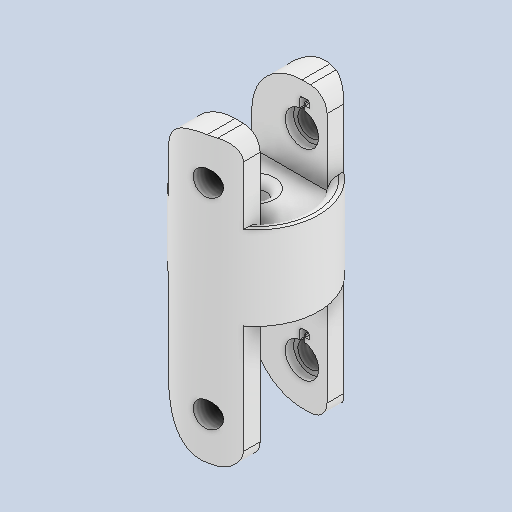
# Autodesk Inventor part: Thumb_1
Saved by Autodesk Inventor 2022 (Build 260153000, 153)
## iProperties
Created: 2023-01-15
Part Number: Thumb_1
Material: ABS Plastic
Document SubType Name: Modeling
Designer: 48735
Density: 1.06 g/cm^3
Appearance: Smooth - White
Author: 48735
Autodesk Inventor part; units mm, degrees
ref_plane "YZ Plane" through (0, 0, 0) normal (1, 0, 0) x (0, 1, 0)
ref_plane "XZ Plane" through (0, 0, 0) normal (0, 1, 0) x (-1, 0, 0)
ref_plane "XY Plane" through (0, 0, 0) normal (0, 0, 1) x (1, 0, 0)
sketch "Sketch1" plane through (0, 0, 0) normal (0, 1, 0) x (-1, 0, 0)
  circle A0 centre (0, 0) radius 7.5
  line L0 (0, -4) -> (6.3443, -4)
  line L1 (0, -4) -> (-6.3443, -4)
  line L2 (0, 4) -> (-6.3443, 4)
  line L3 (0, 4) -> (6.3443, 4)
  line L4 (7.5, 0) -> (4.5, 0)
  line L5 (4.5, 0) -> (4.5, 6)
  line L6 (4.5, 0) -> (4.5, -6)
  line L7 (-7.5, 0) -> (-4.5, 0)
  line L8 (-4.5, 0) -> (-4.5, 6)
  line L9 (-4.5, 0) -> (-4.5, -6)
  point P0 (-4.5, -4)
  point P1 (4.5, -4)
  point P2 (-4.5, 4)
  point P3 (4.5, 4)
  dimension "d5" = 3
  dimension "d6" = 3
  constraints: 20 end point, 5 point on line, 2 parallel, 2 perpendicular, 1 coincident, 12 other
  measures "d5" distance of L4.start L4.end
  measures "d6" distance of L7.start L7.end
extrude "Extrusion1" add sketch "Sketch1" along normal blind 15 contours L5 L3 L2 L8 A0 | A0 L9 L1 L0 L6
sketch "Sketch2" plane through (0, 15, 0) normal (0, 1, 0) x (1, 0, 0)
  circle A0 centre (0, 0) radius 7.5
  circle A1 centre (0, 0) radius 1.25
  dimension "d7" = 2.5
  constraints: 2 centre point, 2 coincident
  measures "d7" diameter of A1
extrude "Extrusion2" add sketch "Sketch2" along normal blind 10
sketch "Sketch3" plane through (-4.5, 0, -4) normal (0, 0, 1) x (1, 0, 0)
  circle A0 centre (3.25, 12.5) radius 1.25
  point P0 (4.5, 0)
  constraints: 1 centre point
extrude "Extrusion3" add sketch "Sketch3" along normal blind 4
chamfer "Chamfer1" distance 0.25 distance2 1.25 1 edges at (-2.5, 12.5, 0) measured on face at (-0.9381, 12.7763, 0)
sketch "Sketch4" plane through (4.5, 0, 4) normal (0, 0, -1) x (-1, 0, 0)
  circle A0 centre (5.75, 12.5) radius 1.25
  point P0 (4.5, 0)
  constraints: 1 centre point
extrude "Extrusion4" add sketch "Sketch4" along normal blind 4
fillet "Fillet1" radius 6 2 edges at (-4.5, 0, 5) (-4.5, 0, -5)
fillet "Fillet2" radius 2 2 edges at (4.5, 0, 5) (4.5, 0, -5)
chamfer "Chamfer2" distance 1 angle 45 1 edges at (-7.5, 15, 0)
chamfer "Chamfer3" distance 0.25 distance2 1.25 1 edges at (0, 12.5, 0) measured on face at (-2.3949, 12.3205, 0)
sketch "Sketch5" plane through (4.5, 15, 4) normal (0, 0, -1) x (-1, 0, 0)
  arc A0 (3, -15) -> (9, -9) centre (3, -9) ccw projected
  line L0 (3, -15) -> (3, -10)
  point P0 (4.5, -15)
  dimension "d29" = 5
  constraints: 2 end point, 1 vertical
  measures "d29" distance of L0.start L0.end
hole "Hole1" at (1.5, 5, 4) direction (0, 0, 1) diameter 3 depth 5 counterbore diameter 4 counterbore depth 1
sketch "Sketch6" plane through (-4.5, 15, -4) normal (0, 0, 1) x (1, 0, 0)
  circle A0 centre (6, -10) radius 1.75 projected
  line L0 (6, -10) -> (7.75, -10)
  point P0 (4.5, -15)
  constraints: 2 end point, 1 horizontal, 1 horizontal alignment, 1 other
hole "Hole2" at (1.5, 5, -4) direction (0, 0, -1) diameter 3 depth 5 tip angle 118 counterbore diameter 4 counterbore depth 1
sketch "Sketch7" plane through (4.5, 15, 4) normal (0, 0, -1) x (-1, 0, 0)
  circle A0 centre (3, -10) radius 1.75 projected
  line L0 (2.75, -7.25) -> (2.75, -10)
  line L1 (2.75, -10) -> (3, -10)
  line L2 (3, -10) -> (3.25, -10)
  line L3 (3.25, -10) -> (3.25, -7)
  arc A1 (3.25, -7) -> (3, -6.75) centre (3, -7) ccw
  line L4 (3, -6.75) -> (2.5, -6.75)
  line L5 (2.5, -6.75) -> (2.375, -6.75)
  arc A2 (2.375, -6.75) -> (2.125, -7) centre (2.375, -7) ccw
  line L6 (2.125, -7) -> (2.125, -7.5)
  line L7 (2.125, -7.5) -> (2.625, -7.5)
  line L8 (2.625, -7.5) -> (2.625, -7.25)
  line L9 (2.625, -7.25) -> (2.75, -7.25)
  circle A3 centre (3, -10) radius 1.75
  line L10 (2.75, -7.25) -> (2.75, -10)
  line L11 (2.75, -10) -> (3, -10)
  line L12 (3, -10) -> (3.25, -10)
  line L13 (3.25, -10) -> (3.25, -7)
  arc A4 (3.25, -7) -> (3, -6.75) centre (3, -7) ccw
  line L14 (3, -6.75) -> (2.5, -6.75)
  line L15 (2.5, -6.75) -> (2.375, -6.75)
  arc A5 (2.375, -6.75) -> (2.125, -7) centre (2.375, -7) ccw
  line L16 (2.125, -7) -> (2.125, -7.5)
  line L17 (2.125, -7.5) -> (2.625, -7.5)
  line L18 (2.625, -7.5) -> (2.625, -7.25)
  line L19 (2.625, -7.25) -> (2.75, -7.25)
  point P0 (4.5, -15)
  point P1 (4.5, -15)
  constraints: 40 end point, 8 perpendicular, 8 point on circle, 6 tangent, 5 centre point, 4 horizontal, 2 point on line, 2 vertical
sketch "Sketch8" plane through (-4.5, 15, -4) normal (0, 0, 1) x (1, 0, 0)
  circle A0 centre (6, -10) radius 1.75
  line L0 (5.75, -8.2679) -> (5.75, -10)
  line L1 (5.75, -10) -> (6, -10)
  line L2 (6, -10) -> (6.25, -10)
  line L3 (6.25, -10) -> (6.25, -7.25)
  line L4 (5.75, -7.25) -> (5.75, -10)
  line L5 (5.75, -10) -> (6, -10)
  line L6 (6, -10) -> (6.25, -10)
  line L7 (6.25, -10) -> (6.25, -7.25)
  circle A1 centre (6, -10) radius 1.75 projected
  circle A2 centre (6, -10) radius 1.75
  line L8 (6.25, -7.25) -> (6.25, -10)
  line L9 (6.25, -10) -> (6, -10)
  line L10 (6, -10) -> (5.75, -10)
  line L11 (5.75, -10) -> (5.75, -7)
  line L12 (6, -6.75) -> (6.5, -6.75)
  line L13 (6.5, -6.75) -> (6.625, -6.75)
  arc A3 (6.875, -7) -> (6.625, -6.75) centre (6.625, -7) ccw
  line L14 (6.875, -7) -> (6.875, -7.5)
  line L15 (6.875, -7.5) -> (6.375, -7.5)
  line L16 (6.375, -7.5) -> (6.375, -7.25)
  line L17 (6.375, -7.25) -> (6.25, -7.25)
  line L18 (6.25, -7.25) -> (6.25, -10)
  line L19 (6.25, -10) -> (6, -10)
  line L20 (6, -10) -> (5.75, -10)
  line L21 (5.75, -10) -> (5.75, -7)
  arc A4 (6, -6.75) -> (5.75, -7) centre (6, -7) ccw
  line L22 (6, -6.75) -> (6.5, -6.75)
  line L23 (6.5, -6.75) -> (6.625, -6.75)
  arc A5 (6.875, -7) -> (6.625, -6.75) centre (6.625, -7) ccw
  line L24 (6.875, -7) -> (6.875, -7.5)
  line L25 (6.875, -7.5) -> (6.375, -7.5)
  line L26 (6.375, -7.5) -> (6.375, -7.25)
  line L27 (6.375, -7.25) -> (6.25, -7.25)
  point P0 (4.5, -15)
  point P1 (4.5, -15)
  point P2 (4.5, -15)
  point P3 (6.25, -8.2679)
  constraints: 56 end point, 6 point on circle, 4 centre point, 4 perpendicular, 4 point on line, 3 other
extrude "Extrusion5" cut sketch "Sketch7" against normal blind 1 contours L3 L2 L1 L0 A0 | A0 L0 L9 L8 L7 L6 A2 L5 L4 A1 L3 picked at (3.1667, -9.4226)
extrude "Extrusion6" cut sketch "Sketch8" against normal blind 1 contours L4 L11 A4 L12 L13 A3 L14 L15 L16 L17 L3 A0
sketch "Sketch9" plane through (0, 25, 0) normal (0, 1, 0) x (1, 0, 0)
  circle A0 centre (0, 0) radius 7.5
  line L0 (-0.5, -4) -> (3.5, -4) projected
  arc A1 (4.5, -6) -> (4.5, 6) centre (0, 0) ccw projected
  line L1 (-2.5, -4) -> (0, -4) projected
  line L2 (3.5, 4) -> (-0.5, 4) projected
  line L3 (1.5, 4) -> (-4.5, 4) projected
  arc A2 (-4.5, 6) -> (-4.5, -6) centre (0, 0) ccw projected
  line L4 (-7.5, 0) -> (-4.5, 0)
  line L5 (-4.5, -6) -> (-4.5, -4) projected
  line L6 (-4.5, -4) -> (-4.5, -6)
  line L7 (-4.5, -6) -> (-4.5, -4)
  line L8 (-4.5, 4) -> (-4.5, 6) projected
  line L9 (-4.5, 4) -> (-4.5, 6)
  line L10 (4.5, 6) -> (4.5, 4) projected
  line L11 (4.5, 6) -> (4.5, 4)
  line L12 (4.5, -6) -> (4.5, -4) projected
  line L13 (4.5, -4) -> (4.5, -6)
  line L14 (-4.5, 4) -> (4.5, 4)
  line L15 (4.5, -4) -> (4.5, -6) projected
  line L16 (4.5, -4) -> (-4.5, -4)
  point P0 (1.25, -4)
  point P1 (1.75, -4)
  point P2 (1.75, 4)
  point P3 (1.25, 4)
  point P4 (3.5, 4)
  constraints: 16 end point, 4 equal length, 1 centre point, 1 coincident, 1 horizontal, 1 perpendicular, 1 point on line, 2 other
extrude "Extrusion7" add sketch "Sketch9" along normal blind 9 contours L10 L14 L2 L3 L8 A0 | A0 L5 L16 L1 L0 L12
fillet "Fillet3" radius 6 2 edges at (-4.5, 34, -5) (-4.5, 34, 5)
fillet "Fillet4" radius 2 2 edges at (4.5, 34, 5) (4.5, 34, -5)
sketch "Sketch10" plane through (4.5, 25, 4) normal (0, 0, -1) x (-1, 0, 0)
  line L0 (2, 9) -> (3, 9) projected
  line L1 (3, 9) -> (3, 4)
  point P0 (4.5, -25)
  dimension "d61" = 5
  constraints: 2 end point, 1 vertical
  measures "d61" distance of L0.end L1.end
hole "Hole3" at (1.5, 29, 4) direction (0, 0, 1) diameter 3 depth 5 counterbore diameter 4 counterbore depth 1
sketch "Sketch11" plane through (-4.5, 25, -4) normal (0, 0, 1) x (1, 0, 0)
  line L0 (6, 9) -> (6, 4)
  point P0 (4.5, -25)
  dimension "d69" = 5
  constraints: 2 end point, 1 vertical
  measures "d69" distance of L0.start L0.end
hole "Hole4" at (1.5, 29, -4) direction (0, 0, -1) diameter 3 depth 5 counterbore diameter 4 counterbore depth 1
chamfer "Chamfer4" distance 1 angle 45 1 edges at (-7.5, 25, 0)
fillet "Fillet5" radius 1 1 edges at (-1.25, 25, 0)
fillet "Fillet6" radius 1 1 edges at (-1.25, 15, 0)
sketch "Sketch12" plane through (4.5, 25, 4) normal (0, 0, -1) x (-1, 0, 0)
  circle A0 centre (3, 4.0015) radius 1.75
  line L0 (2.75, 6.7515) -> (2.75, 4.0015)
  line L1 (2.75, 4.0015) -> (3, 4.0015)
  line L2 (3, 4.0015) -> (3.25, 4.0015)
  line L3 (3.25, 4.0015) -> (3.25, 7.0015)
  arc A1 (3.25, 7.0015) -> (3, 7.2515) centre (3, 7.0015) ccw
  line L4 (3, 7.2515) -> (2.5, 7.2515)
  line L5 (2.5, 7.2515) -> (2.375, 7.2515)
  arc A2 (2.375, 7.2515) -> (2.125, 7.0015) centre (2.375, 7.0015) ccw
  line L6 (2.125, 7.0015) -> (2.125, 6.5015)
  line L7 (2.125, 6.5015) -> (2.625, 6.5015)
  line L8 (2.625, 6.5015) -> (2.625, 6.7515)
  line L9 (2.625, 6.7515) -> (2.75, 6.7515)
  circle A3 centre (3, 4.0015) radius 1.75
  line L10 (2.75, 6.7515) -> (2.75, 4.0015)
  line L11 (2.75, 4.0015) -> (3, 4.0015)
  line L12 (3, 4.0015) -> (3.25, 4.0015)
  line L13 (3.25, 4.0015) -> (3.25, 7.0015)
  arc A4 (3.25, 7.0015) -> (3, 7.2515) centre (3, 7.0015) ccw
  line L14 (3, 7.2515) -> (2.5, 7.2515)
  line L15 (2.5, 7.2515) -> (2.375, 7.2515)
  arc A5 (2.375, 7.2515) -> (2.125, 7.0015) centre (2.375, 7.0015) ccw
  line L16 (2.125, 7.0015) -> (2.125, 6.5015)
  line L17 (2.125, 6.5015) -> (2.625, 6.5015)
  line L18 (2.625, 6.5015) -> (2.625, 6.7515)
  line L19 (2.625, 6.7515) -> (2.75, 6.7515)
  point P0 (4.5, -25)
  point P1 (4.5, -15)
  point P2 (4.5, -15)
  constraints: 40 end point, 8 perpendicular, 8 point on circle, 6 centre point, 6 tangent, 4 horizontal, 2 point on line, 2 vertical
sketch "Sketch13" plane through (-4.5, 25, -4) normal (0, 0, 1) x (1, 0, 0)
  circle A0 centre (6, 3.9996) radius 1.75
  line L0 (5.75, 5.7317) -> (5.75, 3.9996)
  line L1 (5.75, 3.9996) -> (6, 3.9996)
  line L2 (6, 3.9996) -> (6.25, 3.9996)
  line L3 (6.25, 3.9996) -> (6.25, 6.7496)
  line L4 (5.75, 6.7496) -> (5.75, 3.9996)
  line L5 (5.75, 3.9996) -> (6, 3.9996)
  line L6 (6, 3.9996) -> (6.25, 3.9996)
  line L7 (6.25, 3.9996) -> (6.25, 6.7496)
  circle A1 centre (6, 3.9996) radius 1.75
  line L8 (6.25, 3.9996) -> (6, 3.9996)
  line L9 (6.25, 3.9996) -> (6, 3.9996)
  line L10 (6, 3.9996) -> (5.75, 3.9996)
  line L11 (6, 3.9996) -> (5.75, 3.9996)
  line L12 (6.875, 6.4996) -> (6.375, 6.4996)
  line L13 (6.875, 6.4996) -> (6.375, 6.4996)
  line L14 (6.25, 6.7496) -> (6.25, 3.9996)
  line L15 (6.25, 6.7496) -> (6.25, 3.9996)
  line L16 (6.375, 6.7496) -> (6.25, 6.7496)
  line L17 (6.375, 6.7496) -> (6.25, 6.7496)
  line L18 (6.375, 6.4996) -> (6.375, 6.7496)
  line L19 (6.375, 6.4996) -> (6.375, 6.7496)
  line L20 (5.75, 3.9996) -> (5.75, 6.9996)
  line L21 (5.75, 3.9996) -> (5.75, 6.9996)
  line L22 (6, 7.2496) -> (6.5, 7.2496)
  line L23 (6, 7.2496) -> (6.5, 7.2496)
  line L24 (6.5, 7.2496) -> (6.625, 7.2496)
  arc A2 (6.875, 6.9996) -> (6.625, 7.2496) centre (6.625, 6.9996) ccw
  arc A3 (6.875, 6.9996) -> (6.625, 7.2496) centre (6.625, 6.9996) ccw
  arc A4 (6, 7.2496) -> (5.75, 6.9996) centre (6, 6.9996) ccw
  line L25 (6.5, 7.2496) -> (6.625, 7.2496)
  line L26 (6.875, 6.9996) -> (6.875, 6.4996)
  line L27 (6.875, 6.9996) -> (6.875, 6.4996)
  circle A5 centre (6, 3.9996) radius 1.75
  point P0 (4.5, -25)
  point P1 (4.5, -15)
  point P2 (4.5, -15)
  point P3 (4.5, -15)
  point P4 (6, -6.75)
  point P5 (5.75, -7)
  point P6 (5.75, -7.25)
  point P7 (5.75, -8.2679)
  point P8 (6.25, -8.2679)
  point P9 (6, 7.2496)
  point P10 (5.75, 6.9996)
  point P11 (5.75, 6.7496)
  point P12 (5.75, 5.7317)
  point P13 (6.25, 5.7317)
  constraints: 56 end point, 6 point on circle, 5 centre point, 4 perpendicular, 4 point on line, 3 other
extrude "Extrusion8" cut sketch "Sketch13" against normal blind 1 contours L4 L20 A4 L22 L24 A2 L26 L12 L18 L16 L3 A0
extrude "Extrusion9" cut sketch "Sketch12" against normal blind 1 contours L3 L2 L1 L0 A0 | A0 L0 L9 L8 L7 L6 A2 L5 L4 A1 L3 picked at (3.1667, 4.5789)
sketch "Sketch14" plane through (0, 25, 0) normal (0, 1, 0) x (1, 0, 0)
  circle A0 centre (0, 0) radius 1.25 projected
  line L0 (4.5, -4) -> (4.5, -6) projected
  circle A1 centre (0, 0) radius 6.0208
  line L1 (3.25, 5.0683) -> (3.25, 5.0683)
  line L2 (3.5, 5) -> (3.5, 4) projected
  line L3 (-4.5, -6) -> (-4.5, -4) projected
  line L4 (-4.5, -4) -> (4.5, -4)
  line L5 (0, -1.25) -> (-2.5, -1.25) projected
  circle A2 centre (0, 0) radius 1.25
  line L6 (4.5, 4) -> (4.5, 6) projected
  line L7 (-4.5, 4.6904) -> (-4.5, 4) projected
  line L8 (4.5, 4) -> (-4.5, 4)
  constraints: 6 end point, 3 point on circle, 2 coincident, 2 perpendicular, 2 vertical alignment, 1 centre point, 1 horizontal, 2 other
extrude "Extrusion10" cut sketch "Sketch14" against normal blind 1 contours A1 L4 L8
fillet "Fillet7" radius 1 3 edges at (-1.25, 24, 0) (6.0208, 25, 0) (-6.0208, 25, 0)
thread "Thread1" size "M2.5x0.45" class "6H" standard "ANSI Metric M Profile" length 6
thread "Thread2" size "M2.5x0.45" class "6H" standard "ANSI Metric M Profile" length 6
thread "Thread3" size "M2.5x0.45" class "6H" standard "ANSI Metric M Profile" length 6
thread "Thread4" size "M2.5x0.45" class "6H" standard "ANSI Metric M Profile" length 6
body "Solid1"
